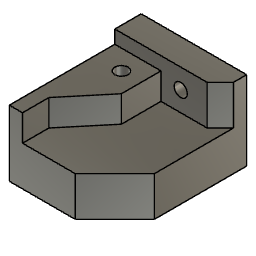
1) (Autodesk Fusion 360 design; units mm, degrees)
Autodesk Fusion 360 part; units mm, degrees
sketch "Sketch1" plane through (0, 0, 0) normal (0, 0, 1) x (1, 0, 0)
  line L0 (0, 0) -> (160, 0)
  line L1 (160, 0) -> (160, -200)
  line L2 (160, -200) -> (0, -200)
  line L3 (0, -200) -> (0, 0)
  dimension "d1" = 160
  dimension "d2" = 200
  constraint horizontal L0
  constraint vertical L1
  constraint horizontal L2
  constraint vertical L3
  constraint coincident L0.start L3.end
  measures "d1" distance of L0.start L0.end
  measures "d2" distance of L0.start L2.end
extrude "Extrude1" add sketch "Sketch1" along normal blind 120
chamfer "Chamfer1" distance 60 angle 45 1 edges at (160, -200, 60)
sketch "Sketch2" plane through (0, 0, 120) normal (0, 0, 1) x (-1, 0, 0)
  line L0 (-100, 200) -> (-160, 140)
  line L1 (-160, 140) -> (-160, 0)
  line L2 (-160, 0) -> (0, 0)
  line L3 (0, 0) -> (0, 200)
  line L4 (0, 200) -> (-100, 200)
  line L5 (0, 200) -> (-160, 200)
  line L6 (-160, 200) -> (-160, 40)
  line L7 (-160, 40) -> (0, 40)
  line L8 (0, 40) -> (0, 200)
  constraint horizontal L5
  constraint vertical L6
  constraint horizontal L7
  constraint vertical L8
  constraint coincident L1 L6.end
  constraint coincident L3.end L4.start
extrude "Extrude2" cut sketch "Sketch2" along normal mid plane 40 contours L0 L1 L3 L4 L5 L6 L7 L8
sketch "Sketch3" plane through (0, 0, 100) normal (0, 0, 1) x (-1, 0, 0)
  line L0 (0, 40) -> (0, 200)
  line L1 (0, 200) -> (-100, 200)
  line L2 (-100, 200) -> (-160, 140)
  line L3 (-160, 140) -> (-160, 40)
  line L4 (-160, 40) -> (0, 40)
  line L5 (-20, 200) -> (-140, 200)
  line L6 (-140, 200) -> (-140, 160)
  line L7 (-140, 160) -> (-20, 160)
  line L8 (-20, 160) -> (-20, 200)
  line L9 (-70, 40) -> (-160, 40)
  line L10 (-160, 40) -> (-160, 100)
  line L11 (-160, 100) -> (-70, 100)
  line L12 (-70, 100) -> (-70, 40)
  line L13 (-20, 160) -> (-70, 100)
  line L14 (-140, 160) -> (-160, 140)
  line L15 (-160, 100) -> (-160, 140)
  constraint horizontal L5
  constraint vertical L6
  constraint horizontal L7
  constraint vertical L8
  constraint coincident L2 L6.end
  constraint coincident L1 L5.start
  constraint horizontal L9
  constraint vertical L10
  constraint horizontal L11
  constraint vertical L12
  constraint coincident L3 L10.end
  constraint coincident L4 L9.start
  constraint coincident L2.end L3.start
extrude "Extrude3" cut sketch "Sketch3" along normal mid plane 80 contours L3 L4 L9 L10 L11 L12 | L1 L2 L5 L7 L8 | L2 L3 L7 L11 L13 L14 L15
chamfer "Chamfer2" distance 20 angle 45 1 edges at (160, -40, 90)
sketch "Sketch4" plane through (0, 0, 100) normal (0, 0, 1) x (-1, 0, 0)
  line L0 (-20, 200) -> (-20, 160)
  line L1 (-20, 160) -> (-70, 100)
  line L2 (-70, 100) -> (-70, 40)
  line L3 (-70, 40) -> (0, 40)
  line L4 (0, 40) -> (0, 200)
  line L5 (0, 200) -> (-20, 200)
  circle A0 centre (-40, 70) radius 10
  dimension "d11" = 20
  measures "d11" diameter of A0
extrude "Extrude4" cut sketch "Sketch4" along normal blind 0 and the other way blind 100 contours A0
sketch "Sketch5" plane through (0, -40, 0) normal (0, -1, 0) x (1, 0, 0)
  line L0 (140, 60) -> (140, 120)
  line L1 (140, 120) -> (0, 120)
  line L2 (0, 120) -> (0, 100)
  line L3 (0, 100) -> (70, 100)
  line L4 (70, 100) -> (70, 60)
  line L5 (70, 60) -> (140, 60)
  circle A0 centre (100, 90) radius 10
  dimension "d16" = 20
  measures "d16" diameter of A0
extrude "Extrude5" cut sketch "Sketch5" along normal blind 0 and the other way blind 40 contours A0
